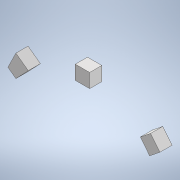
# Autodesk Inventor part: Part17
Saved by Autodesk Inventor 2022.3 (Build 263350000, 350)
## iProperties
Created: 2022-11-17
Part Number: Part17
Material: PET Plastic
Document SubType Name: Modeling
Designer: komputer
Density: 1.541 g/cm^3
Appearance: Polycarbonate - Clear
Author: komputer
Autodesk Inventor part; units mm, degrees
ref_plane "YZ Plane" through (0, 0, 0) normal (1, 0, 0) x (0, 1, 0)
ref_plane "XZ Plane" through (0, 0, 0) normal (0, 1, 0) x (-1, 0, 0)
ref_plane "XY Plane" through (0, 0, 0) normal (0, 0, 1) x (1, 0, 0)
sketch "Sketch1" plane through (0, 0, 0) normal (0, 0, 1) x (1, 0, 0)
  line L0 (25, -7) -> (50, -7) projected
  line L1 (50, 45.5218) -> (50, -7) projected
  line L2 (50, 45.5218) -> (11.4158, 45.5218) projected
  line L3 (11.4158, 45.5218) -> (11.4158, 48.5218) projected
  line L4 (11.4158, 48.5218) -> (-11.4158, 48.5218) projected
  line L5 (-11.4158, 48.5218) -> (-11.4158, 45.5218) projected
  line L6 (-11.4158, 45.5218) -> (-50, 45.5218) projected
  line L7 (-50, 45.5218) -> (-50, -7) projected
  line L8 (-50, -7) -> (-25, -7) projected
  line L9 (-25, -7) -> (-25, -24) projected
  line L10 (-25, -24) -> (-32.4371, -24) projected
  line L11 (-32.4371, -24) -> (-32.4371, -28) projected
  line L12 (-32.4371, -28) -> (-25, -28) projected
  line L13 (-25, -28) -> (-25, -35) projected
  line L14 (-25, -35) -> (25, -35) projected
  line L15 (25, -35) -> (25, -28) projected
  line L16 (25, -28) -> (30.7079, -28) projected
  line L17 (30.7079, -28) -> (30.7079, -24) projected
  line L18 (30.7079, -24) -> (25, -24) projected
  line L19 (25, -24) -> (25, -7) projected
  circle A0 centre (-11.4158, 26.1989) radius 1.6 projected
  circle A1 centre (20.9961, 37.6953) radius 1.6 projected
  circle A2 centre (-20.9961, 37.6953) radius 1.6 projected
  circle A3 centre (11.4158, 26.1989) radius 1.6 projected
  line L20 (3.7761, 48.5218) -> (-5.6641, 48.5218)
  line L21 (-5.6641, 48.5218) -> (-5.6641, 39.2953)
  line L22 (-5.6641, 39.2953) -> (3.7761, 39.2953)
  line L23 (3.7761, 39.2953) -> (3.7761, 48.5218)
  line L24 (50, -35) -> (50, 20.7683) projected
  line L25 (50, 20.7683) -> (-50, 20.7683) projected
  line L26 (-50, 20.7683) -> (-50, -35) projected
  line L27 (-50, -35) -> (50, -35) projected
  line L28 (43.2359, 20.7683) -> (50, 26.1989)
  line L29 (43.8636, 33.8422) -> (50, 26.1989)
  line L30 (43.8636, 33.8422) -> (37.0994, 28.4116)
  line L31 (37.0994, 28.4116) -> (43.2359, 20.7683)
  line L32 (-44.7463, 20.7683) -> (-36.6029, 29.3579)
  line L33 (-36.6029, 29.3579) -> (-44.7463, 35.2815)
  line L34 (-44.7463, 35.2815) -> (-50, 24.59)
  line L35 (-44.7463, 20.7683) -> (-50, 24.59)
  point P0 (0, 0)
  constraints: 24 end point, 5 point on line, 4 perpendicular, 3 parallel, 1 horizontal
extrude "Extrusion1" add sketch "Sketch1" along normal blind 8 contours L28 L31 L30 L29 | L35 L34 L33 L32 | L23 L22 L21 L4
body "Solid1"
